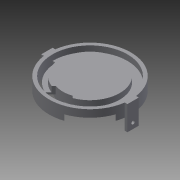
# Autodesk Inventor part: clock_case2
Saved by Autodesk Inventor 2015 SP2 (Build 190223200, 223)
## iProperties
Created: 2016-02-29
Part Number: clock_case2
Material: Generic
Document SubType Name: Modeling
Designer: mca20
Density: 1 g/cm^3
Appearance: Default
Author: mca20
Autodesk Inventor part; units mm, degrees
ref_plane "YZ Plane" through (0, 0, 0) normal (1, 0, 0) x (0, 1, 0)
ref_plane "XZ Plane" through (0, 0, 0) normal (0, 1, 0) x (-1, 0, 0)
ref_plane "XY Plane" through (0, 0, 0) normal (0, 0, 1) x (1, 0, 0)
sketch "Sketch1" plane through (0, 0, 0) normal (0, 1, 0) x (-1, 0, 0)
  circle A0 centre (0, 0) radius 26.25
  circle A1 centre (0, 0) radius 33
  dimension "d0" = 52.5
  dimension "d1" = 66
  constraints: 2 centre point, 2 coincident
  measures "d0" diameter of A0
  measures "d1" diameter of A1
extrude "Extrusion1" add sketch "Sketch1" along normal blind 1.5
sketch "Sketch2" plane through (0, 1.5, 0) normal (0, 1, 0) x (1, 0, 0)
  circle A0 centre (0, 0) radius 25
  circle A1 centre (0, 0) radius 33 projected
  line L0 (-7.5, -23.8485) -> (-13.6817, -30.0302)
  circle A2 centre (0, 0) radius 33 projected
  line L1 (-7.5, -23.8485) -> (1.2422, -23.8485) construction
  line L2 (7.5, -23.8485) -> (13.6817, -30.0302)
  line L3 (7.5, -23.8485) -> (16.2422, -23.8485) construction
  point P0 (0, -25)
  dimension "d4" = 50
  dimension "d5" = 135
  dimension "d6" = 45
  dimension "d7" = 15
  dimension "d9" = 7.5
  dimension "d10" = 0
  dimension "d66" = 8
  constraints: 8 end point, 5 point on circle, 2 equal length, 2 horizontal, 1 centre point, 1 coincident
  measures "d4" diameter of A0
  measures "d5" angle of L0 L1
  measures "d6" angle of L2 L3
  measures "d7" distance of L2.start L0.start
  measures "d9" horizontal distance of point (0, -25) L2.start
  measures "d10" horizontal distance of point (0, -25) A0.centre
  measures "d66" radial gap between concentric circles of A1 A0
extrude "Extrusion2" cut sketch "Sketch2" against normal blind 1.5 contours A0 L2 A1 L0 picked at (9.3939, -28.7092)
sketch "Sketch3" plane through (0, 1.5, 0) normal (0, 1, 0) x (1, 0, 0)
  circle A0 centre (0, 0) radius 30
  arc A1 (13.6817, -30.0302) -> (-13.6817, -30.0302) centre (0, 0) ccw projected
  line L0 (8.4905, -24.839) -> (13.6817, -30.0302) projected
  line L1 (-30, -0.0025) -> (-33, -0.0025)
  arc A2 (13.6817, -30.0302) -> (-13.6817, -30.0302) centre (0, 0) ccw projected
  line L2 (-30, -0.0025) -> (-27, -0.0025) construction
  line L3 (-10.6624, -27.0109) -> (-13.6817, -30.0302)
  line L4 (13.6817, -30.0302) -> (8.4905, -24.839) projected
  line L5 (11.4008, -27.7493) -> (13.6817, -30.0302)
  line L6 (-8.4905, -24.839) -> (-13.6817, -30.0302) projected
  line L7 (-11.4008, -27.7493) -> (-13.6817, -30.0302)
  line L8 (30, -0.0025) -> (33, 0.0056)
  point P0 (7.5, -26.4575)
  point P1 (-7.5, -26.4575)
  dimension "d13" = 60
  dimension "d14" = 180
  constraints: 12 end point, 7 point on circle, 2 collinear, 1 centre point, 1 coincident, 1 horizontal, 6 other
  measures "d13" diameter of A0
  measures "d14" angle of L1 L2
extrude "Extrusion3" cut sketch "Sketch3" against normal blind 10 contours A0 L3 A1 L1 | L8 A1 L0 A0
sketch "Sketch8" plane through (0, 0, 0) normal (0, -1, 0) x (1, 0, 0)
  circle A0 centre (0, 0) radius 33
  circle A1 centre (0, 0) radius 36
  dimension "d29" = 66
  dimension "d30" = 3
  dimension "d91" = 72
  constraints: 2 centre point, 1 coincident
  measures "d29" diameter of A0
  measures "d30" radial gap between concentric circles of A0 A1
  measures "d91" diameter of A1
extrude "Extrusion8" add sketch "Sketch8" against normal blind 6.5
sketch "Sketch16" plane through (0, 0, 0) normal (0, -1, 0) x (1, 0, 0)
  circle A0 centre (0, 0) radius 26.25
  dimension "d67" = 52.5
  constraints: 1 centre point, 1 coincident
  measures "d67" diameter of A0
extrude "Extrusion13" add sketch "Sketch16" against normal blind 6.5
sketch "Sketch19" plane through (0, 6.5, 0) normal (0, 1, 0) x (1, 0, 0)
  circle A0 centre (0, 0) radius 24
  circle A1 centre (0, 0) radius 33
  line L0 (-7.5, -22.798) -> (-14.3681, -29.6661)
  circle A2 centre (0, 0) radius 32.9624
  line L1 (-7.5, -22.798) -> (2.213, -22.798) construction
  line L2 (7.5, -22.798) -> (14.3681, -29.6661)
  line L3 (7.5, -22.798) -> (17.213, -22.798) construction
  point P0 (0, -24)
  dimension "d70" = 48
  dimension "d71" = 135
  dimension "d72" = 45
  dimension "d73" = 15
  dimension "d74" = 7.5
  dimension "d75" = 0
  dimension "d76" = 9
  dimension "d138" = 66
  constraints: 8 end point, 5 point on circle, 3 centre point, 3 coincident, 2 equal length, 2 horizontal
  measures "d70" diameter of A0
  measures "d71" angle of L0 L1
  measures "d72" angle of L2 L3
  measures "d73" distance of L2.start L0.start
  measures "d74" horizontal distance of point (0, -24) L2.start
  measures "d75" horizontal distance of point (0, -24) A0.centre
  measures "d76" radial gap between concentric circles of A1 A0
  measures "d138" diameter of A1
extrude "Extrusion14" cut sketch "Sketch19" against normal blind 6.5 contours A0 L2 A2 L0 picked at (9.7463, -28.1973)
sketch "Sketch20" plane through (0, 0, 0) normal (0, -1, 0) x (1, 0, 0)
  circle A0 centre (0, 0) radius 36 projected
  circle A1 centre (0, 0) radius 33
  dimension "d81" = 72
  dimension "d82" = 3
  dimension "d134" = 66
  constraints: 1 centre point
  measures "d81" diameter of A0
  measures "d82" radial gap between concentric circles of A0 A1
  measures "d134" diameter of A1
extrude "Extrusion15" add sketch "Sketch20" along normal blind 5
thread "Thread1" size "M68x6" class "6H" standard "ANSI Metric M Profile" length 5 offset 6.5
sketch "Sketch21" plane through (0, 0, 0) normal (0, -1, 0) x (1, 0, 0)
  circle A0 centre (0, 0) radius 22.5
  circle A1 centre (0, 0) radius 23.5
  dimension "d87" = 45
  dimension "d88" = 1
  constraints: 2 centre point, 1 coincident
  measures "d87" diameter of A0
  measures "d88" radial gap between concentric circles of A0 A1
extrude "Extrusion16" add sketch "Sketch21" along normal blind 4
sketch "Sketch23" plane through (0, 0, 0) normal (0, -1, 0) x (1, 0, 0)
  circle A0 centre (0, 0) radius 22.5 projected
  line L0 (22.5, 0) -> (0, 22.5)
  line L1 (0, 22.5) -> (20.147, 42.647)
  line L2 (22.5, 0) -> (42.647, 20.147)
  line L3 (42.647, 20.147) -> (20.147, 42.647)
  constraints: 8 end point, 2 perpendicular, 2 point on circle, 1 point on line
extrude "Extrusion17" cut sketch "Sketch23" along normal blind 5 contours A0 L1 L3 L2
sketch "Sketch24" plane through (0, 0, 0) normal (0, -1, 0) x (1, 0, 0)
  circle A0 centre (0, 0) radius 22.5
  dimension "d96" = 45
  constraints: 1 centre point, 1 coincident
  measures "d96" diameter of A0
extrude "Extrusion18" add sketch "Sketch24" along normal blind 2
sketch "Sketch25" plane through (0, -5, 0) normal (0, -1, 0) x (1, 0, 0)
  line L0 (0, -5) -> (0, 5)
  line L1 (0, -5) -> (38, -5)
  line L2 (0, 5) -> (38, 5)
  line L3 (38, -5) -> (38, 5)
  circle A0 centre (0, 0) radius 36 projected
  line L4 (0, -5) -> (-38, -5)
  line L5 (0, 5) -> (-38, 5)
  line L6 (-38, 5) -> (-38, -5)
  point P0 (35.6511, -5)
  point P1 (35.6511, 5)
  point P2 (-35.6511, -5)
  point P3 (-35.6511, 5)
  dimension "d99" = 10
  dimension "d100" = 5
  dimension "d101" = 38
  dimension "d102" = 38
  dimension "d107" = 38
  dimension "d133" = 72
  constraints: 14 end point, 4 horizontal, 4 point on circle, 4 point on line, 1 perpendicular, 1 vertical
  measures "d99" distance of L0.start L0.end
  measures "d100" distance of L0.start point (0, 0)
  measures "d101" distance of L0.start L1.end
  measures "d102" distance of L0.end L2.end
  measures "d107" distance of L0.start L4.end
  measures "d133" diameter of A0
extrude "Extrusion19" add sketch "Sketch25" along normal blind 10 and the other way blind 11.5 contours A0 L2 L3 L1 | L4 L6 L5 A0
sketch "Sketch26" plane through (38, -15, 5) normal (1, 0, 0) x (0, 0, -1)
  circle A0 centre (5, 5) radius 1.5
  line L0 (10, 0) -> (0, 0) projected
  line L1 (0, 10) -> (10, 10) projected
  line L2 (0, 10) -> (0, 0) projected
  line L3 (0, 21.5) -> (10, 21.5) projected
  point P0 (5, 15)
  dimension "d108" = 3
  dimension "d110" = 10
  dimension "d112" = 5
  dimension "d132" = 5
  dimension "d135" = 16.5
  dimension "d136" = 21.5
  dimension "d137" = 5
  constraints: 1 centre point
  measures "d108" diameter of A0
  measures "d110" distance between parallel lines of L0 L1
  measures "d112" distance from line of A0.centre L1
  measures "d132" distance from line of L2 A0.centre
  measures "d135" distance from line of L3 A0.centre
  measures "d136" distance between parallel lines of L3 L0
  measures "d137" distance from line of L0 A0.centre
hole "Hole3" at (38, -10, 0) direction (-1, 0, 0) diameter 3 depth 8 tip angle 118
sketch "Sketch27" plane through (-38, -15, -5) normal (-1, 0, 0) x (0, 0, 1)
  line L0 (10, 0) -> (0, 0) projected
  line L1 (0, 10) -> (10, 10) projected
  circle A0 centre (5, 5) radius 1.5
  line L2 (10, 21.5) -> (10, 0) projected
  line L3 (0, 0) -> (0, 21.5) projected
  point P0 (5, 15)
  dimension "d120" = 10
  dimension "d121" = 3
  dimension "d122" = 5
  dimension "d123" = 10
  dimension "d124" = 5
  constraints: 1 centre point
  measures "d120" distance between parallel lines of L0 L1
  measures "d121" diameter of A0
  measures "d122" distance from line of A0.centre L1
  measures "d123" distance between parallel lines of L2 L3
  measures "d124" distance from line of L3 A0.centre
hole "Hole4" at (-38, -10, 0) direction (1, 0, 0) diameter 3 depth 8 tip angle 118
equation "\"d102\" = d101"
equation "\"d107\" = d101"
body "Solid1"
